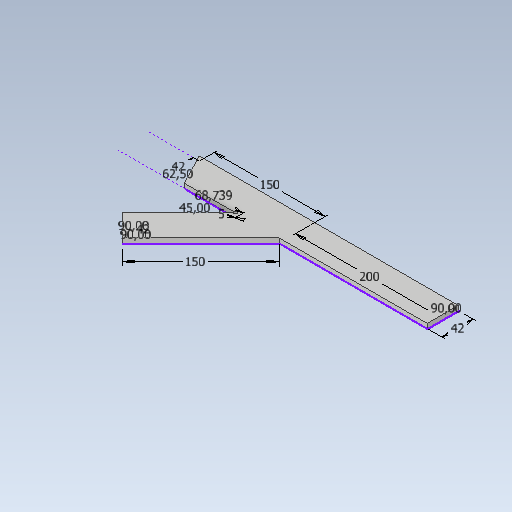
# Autodesk Inventor part: A_Base
Saved by Autodesk Inventor 2020 (Build 240168000, 168)
## iProperties
Created: 2020-12-21
Part Number: A_Base
Material: Generic
Document SubType Name: Modeling
Designer: Dell
Density: 1 g/cm^3
Appearance: Default
Author: Dell
Autodesk Inventor part; units mm, degrees
ref_plane "YZ Plane" through (0, 0, 0) normal (1, 0, 0) x (0, 1, 0)
ref_plane "XZ Plane" through (0, 0, 0) normal (0, 1, 0) x (-1, 0, 0)
ref_plane "XY Plane" through (0, 0, 0) normal (0, 0, 1) x (1, 0, 0)
sketch "Sketch1" plane through (0, 0, 0) normal (0, 1, 0) x (-1, 0, 0)
  line L0 (0, 0) -> (200, 0)
  line L1 (200, 0) -> (350, 0)
  line L2 (350, 0) -> (419.2566, 0) construction
  line L3 (0, 23.5278) -> (0, 0)
  line L4 (0, 0) -> (0, 42)
  line L5 (350, 0) -> (328.1362, 42)
  line L6 (328.1362, 42) -> (417.945, 42) construction
  line L7 (200, 42) -> (306.066, 148.066)
  line L8 (0, 42) -> (200, 42)
  line L9 (261.897, 42) -> (328.1362, 42)
  arc A0 (261.1647, 43.7678) -> (261.897, 42) centre (259.397, 42) ccw
  line L10 (306.066, 148.066) -> (335.7645, 118.3675)
  line L11 (335.7645, 118.3675) -> (261.1647, 43.7678)
  line L12 (0, 0) -> (0, 42)
  line L13 (350, 0) -> (0, 0)
  line L14 (0, 0) -> (0, 42)
  line L15 (0, 42) -> (200, 42)
  line L16 (200, 42) -> (306.066, 148.066)
  line L17 (306.066, 148.066) -> (335.7645, 118.3675)
  line L18 (335.7645, 118.3675) -> (261.1647, 43.7678)
  line L19 (200, 42) -> (259.397, 42) construction
  line L20 (261.897, 42) -> (330, 42) construction
  line L21 (261.897, 42) -> (328.1362, 42)
  dimension "d0" = 200
  dimension "d1" = 150
  dimension "d4" = 42
  dimension "d6" = 62.5
  dimension "d9" = 150
  dimension "d10" = 90
  dimension "d12" = 68.7392
  dimension "d15" = 5
  dimension "d17" = 42
  dimension "d18" = 42
  dimension "d19" = 45
  dimension "d20" = 90
  dimension "d21" = 90
  constraints: 44 end point, 7 collinear, 2 point on circle, 2 point on line, 1 centre point, 1 horizontal
  measures "d0" distance of L0.start L0.end
  measures "d1" distance of L0.end L1.end
  measures "d4" distance of L0.start L4.end
  measures "d6" angle of L6 L5
  measures "d9" distance of L7.start L7.end
  measures "d10" angle of L0 L3
  measures "d12" distance of L19.end L5.end
  measures "d15" diameter of A0
  measures "d17" vertical distance of L1.end L5.end
  measures "d18" distance of L7.end L10.end
  measures "d19" angle of L9 L11
  measures "d20" angle of L10 L11
  measures "d21" angle of L10 L7
extrude "Extrusion1" add sketch "Sketch1" along normal blind 6
body "Solid1"
